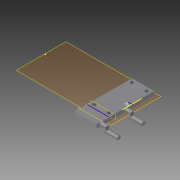
# Autodesk Inventor part: holder
Saved by Autodesk Inventor 2015 (Build 190159000, 159)
## iProperties
Created: 2015-11-09
Part Number: holder
Material: Generic
Document SubType Name: Modeling
Designer: Ross
Density: 1 g/cm^3
Appearance: Default
Author: Ross
Autodesk Inventor part; units mm, degrees
ref_plane "YZ Plane" through (0, 0, 0) normal (1, 0, 0) x (0, 1, 0)
ref_plane "XY Plane" through (0, 0, 0) normal (0, 0, 1) x (1, 0, 0)
sketch "Sketch1" plane through (0, 0, 0) normal (0, 1, 0) x (-1, 0, 0)
  line L0 (70, 0) -> (70, -70)
  line L1 (70, -70) -> (0, -70)
  line L2 (-70, 0) -> (-70, 70)
  line L3 (-70, 70) -> (0, 70)
  line L4 (0, 70) -> (70, 70)
  line L5 (70, 70) -> (70, 0)
  line L6 (0, -70) -> (-70, -70)
  line L7 (-70, -70) -> (-70, 0)
  point P0 (0, 0)
  constraints: 16 end point, 4 perpendicular, 2 point on line, 1 vertical
extrude "Extrusion1" add sketch "Sketch1" along normal blind 3
fillet "Fillet1" radius 5 3 edges at (70, 1.5, 70) (70, 1.5, -70) (-70, 1.5, 70)
fillet "Fillet2" radius 5 1 edges at (-70, 1.5, -70)
ref_plane "Work Plane1" through (65, 0, 65) normal (1, 0, 0) x (0, 0, -1)
sketch "Sketch6" plane through (70, 0, 65) normal (1, 0, 0) x (0, 0, -1)
  line L0 (65, 0) -> (57.2, 0)
  line L1 (130, 0) -> (0, 0) projected
  line L2 (65, 0) -> (72.8, 0)
  line L3 (57.2, 0) -> (57.2, -18)
  line L4 (72.8, 0) -> (72.8, -18)
  line L5 (65, 0) -> (65, -10)
  arc A0 (57.2, -18) -> (72.8, -18) centre (65, -10.2437) ccw
  line L6 (57.2, 0) -> (54.2, 0)
  line L7 (54.2, 0) -> (54.2, -18)
  line L8 (72.8, 0) -> (75.8, 0)
  line L9 (75.8, 0) -> (75.8, -18)
  arc A1 (54.2, -18) -> (75.8, -18) centre (65, -9.0916) ccw
  dimension "d17" = 18
  dimension "d21" = 3
  dimension "d22" = 3
  constraints: 18 end point, 4 point on circle, 4 point on line, 3 perpendicular, 2 centre point, 2 vertical
  measures "d17" distance of L0.end L3.end
  measures "d21" distance of L0.end L6.end
  measures "d22" distance of L2.end L8.end
extrude "Extrusion3" add sketch "Sketch6" against normal blind 18 contours L3 A0 L4 L1 L9 A1 L7
pattern_circular "Circular Pattern1" count 4 over 360 about axis through (0, -10, 0) along (0, 1, 0) of "Extrusion3"
sketch "Sketch8" plane through (0, 3, 0) normal (0, 1, 0) x (1, 0, 0)
  circle A0 centre (58.4636, -19.348) radius 2.5
  point P0 (0, 0)
  dimension "d35" = 5
  constraints: 1 centre point
  measures "d35" diameter of A0
extrude "Extrusion5" cut sketch "Sketch8" against normal blind 3
sketch "Sketch9" plane through (0, 3, 0) normal (0, 1, 0) x (1, 0, 0)
  circle A0 centre (-60.6489, 18.9578) radius 2.5
  point P0 (0, 0)
  dimension "d39" = 5
  constraints: 1 centre point
  measures "d39" diameter of A0
extrude "Extrusion6" cut sketch "Sketch9" against normal blind 3
sketch "Sketch10" plane through (0, 3, 0) normal (0, 1, 0) x (1, 0, 0)
  line L0 (70, -65) -> (70, 65) projected
  line L1 (70, 15.1257) -> (39.2687, 15.1257)
  line L2 (39.2687, 15.1257) -> (39.2687, -15.3197)
  line L3 (39.2687, -15.3197) -> (70, -15.3197)
  line L4 (70, -15.3197) -> (70, 15.1257)
  point P0 (0, 0)
  constraints: 8 end point, 2 parallel, 1 horizontal, 1 perpendicular, 1 point on line
extrude "Extrusion7" add sketch "Sketch10" along normal blind 10
sketch "Sketch11" plane through (0, 3, 0) normal (0, 1, 0) x (1, 0, 0)
  point P0 (0, 0)
sketch "Sketch12" plane through (0, 3, 0) normal (0, 1, 0) x (1, 0, 0)
  line L0 (39.2687, -15.3197) -> (39.2687, -70)
  line L1 (10.8, -70) -> (65, -70) projected
  line L2 (39.2687, -15.3197) -> (39.2687, 15.1257) projected
  line L3 (39.2687, -70) -> (-73.9803, -70)
  line L4 (-73.9803, -70) -> (-73.9803, 75.2408)
  line L5 (-73.9803, 75.2408) -> (39.2687, 75.2408)
  line L6 (39.2687, 75.2408) -> (39.2687, -70)
  point P0 (0, 0)
  constraints: 10 end point, 2 parallel, 1 collinear, 1 horizontal, 1 perpendicular, 1 point on line
extrude "Extrusion8" cut sketch "Sketch12" against normal blind 100
sketch "Sketch13" plane through (0, 3, 0) normal (0, 1, 0) x (1, 0, 0)
  line L0 (39.2687, -15.3197) -> (74.5621, -15.3197)
  line L1 (74.5621, -15.3197) -> (74.5621, -76.2104)
  line L2 (74.5621, -76.2104) -> (39.2687, -76.2104)
  line L3 (39.2687, -76.2104) -> (39.2687, -15.3197)
  point P0 (0, 0)
  constraints: 8 end point, 2 parallel, 1 horizontal, 1 perpendicular
extrude "Extrusion9" cut sketch "Sketch13" against normal blind 100
sketch "Sketch14" plane through (0, 3, 0) normal (0, 1, 0) x (1, 0, 0)
  line L0 (39.2687, 15.1257) -> (72.3919, 15.1257)
  line L1 (72.3919, 15.1257) -> (72.3919, 74.5163)
  line L2 (72.3919, 74.5163) -> (39.2687, 74.5163)
  line L3 (39.2687, 74.5163) -> (39.2687, 15.1257)
  point P0 (0, 0)
  constraints: 8 end point, 2 parallel, 1 horizontal, 1 perpendicular
extrude "Extrusion10" cut sketch "Sketch14" against normal blind 100
sketch "Sketch17" plane through (70, -18, 10.8) normal (1, 0, 0) x (0, 0, -1)
  line L0 (-4.5197, 18) -> (-4.5197, 21)
  line L1 (-4.5197, 18) -> (-4.5197, 31) projected
  line L2 (-4.5197, 21) -> (25.9257, 21)
  line L3 (25.9257, 31) -> (25.9257, 18) projected
  line L4 (25.9257, 21) -> (-4.5197, 21)
  line L5 (-4.5197, 21) -> (-4.5197, 31)
  line L6 (-4.5197, 31) -> (25.9257, 31)
  line L7 (25.9257, 31) -> (25.9257, 21)
  point P0 (10.8, 18)
  dimension "d50" = 3
  constraints: 12 end point, 2 parallel, 2 perpendicular, 2 point on line, 1 horizontal
  measures "d50" distance of L0.start L0.end
extrude "Extrusion11" cut sketch "Sketch17" against normal blind 100
sketch "Sketch18" plane through (39.2687, 0, -15.1257) normal (-1, 0, 0) x (0, 0, 1)
  line L0 (0, 3) -> (30.4454, 3)
  line L1 (30.4454, 3) -> (30.4454, 0)
  line L2 (30.4454, 0) -> (0, 0)
  line L3 (0, 0) -> (0, 3)
  point P0 (15.1257, 0)
  constraints: 8 end point, 2 parallel, 1 horizontal, 1 perpendicular
extrude "Extrusion12" cut sketch "Sketch18" against normal blind 13
sketch "Sketch20" plane through (52, 0, 65) normal (-1, 0, 0) x (0, 0, 1)
  line L0 (-72.8, -18) -> (-72.8, 0) projected
  line L1 (-72.8, -9) -> (-57.2, -9)
  line L2 (-57.2, -18) -> (-57.2, 0) projected
  line L3 (-72.8, -18) -> (-72.8, -4)
  arc A0 (-72.8, -18) -> (-57.2, -18) centre (-65, -10.2437) ccw projected
  line L4 (-65, -21.2437) -> (-72.8, -21.2437)
  line L5 (-72.8, -4) -> (-72.8, -0.8)
  line L6 (-65, -21.2437) -> (-65, -3.2437)
  line L7 (-65, -21.2437) -> (-65, -11.2437)
  line L8 (-65, -11.2437) -> (-65, -1.2437)
  line L9 (-65, -1.2437) -> (-65, -0.8)
  arc A1 (-65, -0.8) -> (-72.6527, -4.1368) centre (-65, -11.2437) ccw
  arc A2 (-57.2, -4.2988) -> (-65, -0.8) centre (-65, -11.2437) ccw
  arc A3 (-72.6527, -4.1368) -> (-72.8, -4.2988) centre (-65, -11.2437) ccw
  arc A4 (-57.2, -4.2988) -> (-57.2, -4.2988) centre (-65, -11.2437) ccw
  line L10 (-72.8, -4.2988) -> (-72.8, 0)
  line L11 (-57.2, 0) -> (-57.2, -4.2988)
  line L12 (-57.2, 0) -> (-72.8, 0) projected
  line L13 (-57.2, -4.2988) -> (-57.2, 0)
  line L14 (-72.8, -4.2988) -> (-72.8, 0)
  line L15 (-72.8, 0) -> (-57.2, 0)
  point P0 (-65, 0)
  dimension "d55" = 14
  dimension "d56" = 3.2
  dimension "d57" = 18
  dimension "d58" = 10
  dimension "d59" = 10
  constraints: 26 end point, 9 point on circle, 4 centre point, 4 coincident, 4 point on line, 3 collinear, 2 midpoint, 2 vertical, 1 horizontal, 1 perpendicular, 1 tangent
  measures "d55" distance of L0.start L3.end
  measures "d56" distance of L3.end L5.end
  measures "d57" distance of L4.start L6.end
  measures "d58" distance of L4.start L7.end
  measures "d59" distance of L7.end L8.end
extrude "Extrusion13" add sketch "Sketch20" against normal blind 18 contours L0 L12 L2 A2 A1 A3
sketch "Sketch22" plane through (52.2687, 0, 10.8) normal (0, 1, 0) x (1, 0, 0)
  line L0 (-0.2687, 21.6) -> (0, 21.6)
  line L1 (0, 21.6) -> (0, 0)
  line L2 (0, 0) -> (-0.2687, 0)
  line L3 (-0.2687, 0) -> (-0.2687, 21.6)
  point P0 (-52.2687, 10.8)
  constraints: 8 end point, 2 parallel, 1 horizontal, 1 perpendicular
extrude "Extrusion14" add sketch "Sketch22" along normal blind 3
sketch "Sketch24" plane through (52.2687, 0, -15.1257) normal (-1, 0, 0) x (0, 0, 1)
  line L0 (30.4454, 3) -> (25.9257, 3)
  line L1 (25.9257, 3) -> (25.9257, 0)
  line L2 (25.9257, 0) -> (30.4454, 0)
  line L3 (30.4454, 0) -> (30.4454, 3)
  point P0 (15.1257, 0)
  constraints: 8 end point, 2 parallel, 1 horizontal, 1 perpendicular
extrude "Extrusion16" add sketch "Sketch24" along normal blind 0.3
sketch "Sketch25" plane through (52.2687, 0, -15.1257) normal (-1, 0, 0) x (0, 0, 1)
  line L0 (0, 0) -> (4.3257, 0)
  line L1 (4.3257, 0) -> (4.3257, 3)
  line L2 (4.3257, 3) -> (0, 3)
  line L3 (0, 3) -> (0, 0)
  point P0 (15.1257, 0)
  constraints: 8 end point, 2 parallel, 1 horizontal, 1 perpendicular
extrude "Extrusion17" add sketch "Sketch25" along normal blind 0.27
sketch "Sketch26" plane through (51.9687, 0, -15.1257) normal (-1, 0, 0) x (0, 0, 1)
  line L0 (30.4454, 3) -> (25.9257, 3)
  line L1 (25.9257, 3) -> (25.9257, 0)
  line L2 (25.9257, 0) -> (30.4454, 0)
  line L3 (30.4454, 0) -> (30.4454, 3)
  point P0 (15.1257, 0)
  constraints: 8 end point, 2 parallel, 1 horizontal, 1 perpendicular
extrude "Extrusion18" cut sketch "Sketch26" against normal blind 0.03
sketch "Sketch27" plane through (70, 0, 15.3197) normal (0, 0, 1) x (1, 0, 0)
  line L0 (0, 3) -> (-18, 3)
  line L1 (-18, 3) -> (-18, 0)
  line L2 (-18, 0) -> (0, 0)
  line L3 (0, 0) -> (0, 3)
  point P0 (-70, 0)
  constraints: 8 end point, 2 parallel, 1 horizontal, 1 perpendicular
extrude "Extrusion19" add sketch "Sketch27" along normal blind 3
sketch "Sketch32" plane through (51.9987, 0, -15.1257) normal (-1, 0, 0) x (0, 0, 1)
  line L0 (4.3257, 0) -> (-3, 0)
  line L1 (-3, 0) -> (-3, 3)
  line L2 (-3, 3) -> (4.3257, 3)
  line L3 (4.3257, 3) -> (4.3257, 0)
  point P0 (15.1257, 0)
  constraints: 8 end point, 2 parallel, 1 horizontal, 1 perpendicular
extrude "Extrusion21" cut sketch "Sketch32" against normal blind 30
sketch "Sketch33" plane through (51.9987, 0, -15.1257) normal (-1, 0, 0) x (0, 0, 1)
  line L0 (33.4454, 0) -> (25.9257, 0) projected
  line L1 (25.9257, 3) -> (33.4257, 3)
  line L2 (33.4257, 3) -> (33.4257, 0)
  line L3 (33.4257, 0) -> (25.9257, 0)
  line L4 (25.9257, 0) -> (25.9257, 3)
  point P0 (15.1257, 0)
  dimension "d86" = 7.5
  constraints: 8 end point, 2 parallel, 1 horizontal, 1 perpendicular, 1 point on line
  measures "d86" distance of L2.end L3.end
extrude "Extrusion22" add sketch "Sketch33" against normal blind 18
sketch "Sketch34" plane through (52, 3, -10.8) normal (0, 1, 0) x (1, 0, 0)
  line L0 (18, -29.1197) -> (18, -26.1197)
  line L1 (18, -29.1197) -> (18, -21.6) projected
  line L2 (18, -26.1197) -> (-0.0013, -26.1197)
  line L3 (-0.0013, -29.1) -> (-0.0013, -21.6) projected
  line L4 (-0.0013, -26.1197) -> (2.9987, -26.1197)
  line L5 (18, -26.1197) -> (15, -26.1197)
  circle A0 centre (15, -26.1197) radius 1.5
  circle A1 centre (2.9987, -26.1197) radius 1.5
  point P0 (-52, -10.8)
  dimension "d89" = 3
  dimension "d90" = 3
  dimension "d91" = 3
  dimension "d92" = 3
  dimension "d93" = 3
  constraints: 8 end point, 4 point on line, 2 centre point, 2 coincident, 1 perpendicular
  measures "d89" distance of L0.start L0.end
  measures "d90" distance of L2.end L4.end
  measures "d91" distance of L0.end L5.end
  measures "d92" diameter of A0
  measures "d93" diameter of A1
extrude "Extrusion23" cut sketch "Sketch34" against normal blind 18
sketch "Sketch35" plane through (70, -18, -10.8) normal (0, 0, -1) x (-1, 0, 0)
  line L0 (18, 21) -> (0, 21)
  line L1 (0, 21) -> (0, 18)
  line L2 (0, 18) -> (18, 18)
  line L3 (18, 18) -> (18, 21)
  point P0 (70, 18)
  constraints: 8 end point, 2 parallel, 1 horizontal, 1 perpendicular
extrude "Extrusion24" add sketch "Sketch35" along normal blind 7.5
mirror "Mirror1" about plane through (0, 0, 0) normal (0, 0, 1) of "Extrusion23"
sketch "Sketch36" plane through (52, 3, 18.3197) normal (0, 1, 0) x (1, 0, 0)
  line L0 (18, 26.1197) -> (18, 10.5197) projected
  line L1 (18, 18.3197) -> (15, 18.3197)
  point P0 (-52, 18.3197)
  dimension "d98" = 3
  constraints: 2 end point, 1 horizontal, 1 midpoint
  measures "d98" distance of L1.start L1.end
sketch "Sketch37" plane through (52, 3, 18.3197) normal (0, 1, 0) x (1, 0, 0)
  line L0 (18, 0) -> (0, 0)
  line L1 (18, 0) -> (9, 0)
  line L2 (0, 0) -> (18, 0) projected
  point P0 (-52, 18.3197)
  constraints: 4 end point, 1 horizontal, 1 midpoint
ref_plane "Work Plane2" through (0, 0, 0) normal (0, 1, 0) x (-1, 0, 0)
sketch "Sketch38" plane through (0, 0, 0) normal (0, 1, 0) x (-1, 0, 0)
  line L0 (-70, -18.3) -> (-51.9987, -18.3)
  line L1 (-51.9987, -18.3) -> (-51.9987, 18.3)
  line L2 (-51.9987, 18.3) -> (-70, 18.3)
  line L3 (-70, 18.3) -> (-70, -18.3)
  point P0 (0, 0)
  constraints: 8 end point, 2 parallel, 1 horizontal, 1 perpendicular
extrude "Extrusion25" cut sketch "Sketch38" against normal blind 30
sketch "Sketch39" plane through (70, 0, 18.3197) normal (0, 0, 1) x (1, 0, 0)
  line L0 (0, 0) -> (-18, 0)
  line L1 (-18, 0) -> (-18, 3)
  line L2 (-18, 3) -> (0, 3)
  line L3 (0, 3) -> (0, 0)
  point P0 (-70, 0)
  constraints: 8 end point, 2 parallel, 1 horizontal, 1 perpendicular
extrude "Extrusion26" add sketch "Sketch39" along normal blind 10
sketch "Sketch40" plane through (70, 0, -18.3) normal (1, 0, 0) x (0, 0, -1)
  line L0 (0, 3) -> (-46.6197, 3) projected
  line L1 (-18.3, 3) -> (-18.3, 0)
  line L2 (0, 0) -> (-29.1, 0) projected
  line L3 (-18.3, 3) -> (-9.3, 3)
  line L4 (-9.3, 3) -> (-9.3, 1.5)
  line L5 (-46.6197, 1.5) -> (-42.6197, 1.5)
  circle A0 centre (-9.3, 1.5) radius 1.5
  circle A1 centre (-42.6197, 1.5) radius 1.5
  dimension "d104" = 9
  dimension "d105" = 4
  constraints: 8 end point, 2 coincident, 2 perpendicular, 2 point on line, 1 centre point, 1 horizontal, 1 tangent, 1 vertical alignment, 2 other
  measures "d104" distance of L1.start L3.end
  measures "d105" distance of L5.start L5.end
ref_plane "Work Plane3" through (70, 0, 24.3197) normal (0, 0, 1) x (1, 0, 0)
sketch "Sketch41" plane through (70, 0, 24.3197) normal (0, 0, 1) x (1, 0, 0)
  line L0 (0, 0) -> (0, 3) projected
  line L1 (0, 1.5) -> (4, 1.5)
  line L2 (4, 1.5) -> (4, -1.5)
  line L3 (4, -1.5) -> (14, -1.5)
  point P0 (-70, 0)
  dimension "d107" = 4
  dimension "d108" = 3
  dimension "d109" = 10
  constraints: 6 end point, 1 horizontal, 1 midpoint, 1 perpendicular, 1 vertical
  measures "d107" distance of L1.start L1.end
  measures "d108" distance of L1.end L2.end
  measures "d109" distance of L2.end L3.end
sweep "Sweep1" add profiles "Sketch40" path "Sketch41" path curves L1 L2 L3 contours A1
ref_plane "Work Plane4" through (70, 0, 14.3197) normal (0, 0, 1) x (1, 0, 0)
mirror "Mirror2" about plane through (70, 0, 14.3197) normal (0, 0, 1) of "Sweep1"
ref_plane "Work Plane5" through (70, 0, 14.3197) normal (0, 0, 1) x (1, 0, 0)
body "Solid1"
